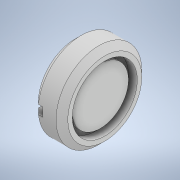
# Autodesk Inventor part: 711127
Saved by Autodesk Inventor 2022 (Build 260153000, 153)
## iProperties
Created: 2021-10-22
Part Number: 711127
Material: Типовые
Document SubType Name: Modeling
Designer: RaNSiD
Density: 1 g/cm^3
Appearance: По умолчанию
Author: RaNSiD
Autodesk Inventor part; units mm, degrees
ref_plane "YZ Plane" through (0, 0, 0) normal (1, 0, 0) x (0, 1, 0)
ref_plane "XZ Plane" through (0, 0, 0) normal (0, 1, 0) x (-1, 0, 0)
ref_plane "XY Plane" through (0, 0, 0) normal (0, 0, 1) x (1, 0, 0)
sketch "Эскиз1" plane through (0, 0, 0) normal (0, 0, 1) x (1, 0, 0)
  line L0 (0, 0) -> (20, 0)
  line L1 (20, 0) -> (20, 25)
  line L2 (16, 29) -> (4, 29)
  line L3 (0, 25) -> (0, 0)
  line L4 (4, 29) -> (0, 25)
  line L5 (16, 29) -> (20, 25)
  point P0 (20, 29)
  point P1 (0, 29)
  dimension "d14" = 20
  dimension "d15" = 29
  dimension "d16" = 4
  dimension "d17" = 4
  dimension "d18" = 4
  dimension "d19" = 4
  constraints: 12 end point, 4 point on line, 2 parallel, 1 horizontal, 1 perpendicular
  measures "d14" distance of point (0, 29) point (20, 29)
  measures "d15" distance of point (20, 29) L0.end
  measures "d16" distance of L2.end point (0, 29)
  measures "d17" distance of L3.start point (0, 29)
  measures "d18" distance of L2.start point (20, 29)
  measures "d19" distance of L1.end point (20, 29)
revolve "Вращение3" add sketch "Эскиз1" angle 360 about axis through (0, 0, 0) along (1, 0, 0)
sketch "Эскиз3" plane through (0, 0, 0) normal (0, 0, 1) x (1, 0, 0)
  line L0 (20, -25) -> (20, 25) construction
  line L1 (20, 0) -> (20, 22)
  line L2 (14, 22) -> (20, 22)
  line L3 (14, 22) -> (14, 19)
  line L4 (14, 19) -> (17, 19)
  line L5 (17, 19) -> (17, 0)
  line L6 (17, 0) -> (20, 0)
  point P0 (0, 0)
  dimension "d21" = 22
  dimension "d22" = 19
  dimension "d23" = 6
  dimension "d24" = 3
  constraints: 12 end point, 4 perpendicular, 1 midpoint, 1 point on line, 1 vertical
  measures "d21" distance of L1.start L1.end
  measures "d22" distance of L4.end L5.end
  measures "d23" distance of L2.start L1.end
  measures "d24" distance between parallel lines of L0 L5
revolve "Вращение4" cut sketch "Эскиз3" angle 360 about axis through (17, 0, 0) along (1, 0, 0)
sketch "Эскиз4" plane through (0, 0, 0) normal (0, 0, 1) x (1, 0, 0)
  line L0 (0, -25) -> (0, 25) construction
  line L1 (0, 3) -> (7, 3)
  line L2 (7, 3) -> (7, -3)
  line L3 (7, -3) -> (0, -3)
  line L4 (0, -3) -> (0, 3)
  point P0 (0, 0)
  point P1 (0, 0)
  point P2 (0, 0)
  dimension "d26" = 7
  dimension "d27" = 6
  constraints: 8 end point, 2 midpoint, 2 parallel, 1 coincident, 1 horizontal, 1 perpendicular, 1 point on line
  measures "d26" distance of L2.end L3.end
  measures "d27" distance of L1.end L2.end
extrude "Выдавливание1" cut sketch "Эскиз4" along normal through all both and the other way through all
equation "\"d17\" = d16"
equation "\"d18\" = d16"
equation "\"d19\" = d18"
